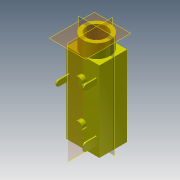
# Autodesk Inventor part: MJ-4535-3
Saved by Autodesk Inventor 2015 SP1 (Build 190203100, 203)
## iProperties
Created: 2015-04-15
Part Number: MJ-4535-3
Material: ABS プラスチック
Document SubType Name: Modeling
Designer: Yamaura
Density: 1.06 g/cm^3
Appearance: 滑らか - 黄
Author: Yamaura
Autodesk Inventor part; units mm, degrees
sketch "スケッチ1" plane through (0, 0, 0) normal (0, 0, 1) x (1, 0, 0)
  circle A0 centre (0, 0) radius 2.5
  circle A1 centre (0, 0) radius 1.8
  dimension "d0" = 5
  dimension "d1" = 3.6
  constraints: 2 centre point, 1 coincident
  measures "d0" diameter of A0
  measures "d1" diameter of A1
extrude "押し出し1" add sketch "スケッチ1" against normal blind 2.5
sketch "スケッチ2" plane through (0, 0, -2.5) normal (0, 0, -1) x (-1, 0, 0)
  line L0 (-3, 2.5) -> (3, 2.5)
  line L1 (3, 2.5) -> (3, -2.5)
  line L2 (3, -2.5) -> (-3, -2.5)
  line L3 (-3, -2.5) -> (-3, 2.5)
  point P0 (0, 0)
  dimension "d4" = 2.5
  dimension "d5" = 5
  dimension "d6" = 3
  dimension "d7" = 6
  constraints: 8 end point, 2 parallel, 1 horizontal, 1 perpendicular
  measures "d4" distance from line of L2 point (0, 0)
  measures "d5" distance of L2.end L0.start
  measures "d6" distance from line of L3 point (0, 0)
  measures "d7" distance of L0.start L0.end
extrude "押し出し2" add sketch "スケッチ2" along normal blind 14.5
sketch "スケッチ3" plane through (-3, -2.5, -2.5) normal (0, -1, 0) x (1, 0, 0)
  circle A0 centre (3, -3.6) radius 0.725
  line L0 (3, 0) -> (6, 0) projected
  circle A1 centre (3, -10.6) radius 0.725
  point P0 (3, 2.5)
  dimension "d10" = 1.45
  dimension "d11" = 3.6
  dimension "d12" = 1.45
  dimension "d13" = 7
  constraints: 2 centre point
  measures "d10" diameter of A0
  measures "d11" distance from line of L0 A0.centre
  measures "d12" diameter of A1
  measures "d13" distance of A1.centre A0.centre
extrude "押し出し3" add sketch "スケッチ3" along normal blind 0.8
sketch "スケッチ4" plane through (-3, -2.5, -2.5) normal (0, -1, 0) x (1, 0, 0)
  line L0 (5.35, -2.2) -> (5.55, -2.2)
  line L1 (5.55, -2.2) -> (5.55, -3.2)
  line L2 (5.55, -3.2) -> (5.35, -3.2)
  line L3 (5.35, -3.2) -> (5.35, -2.2)
  line L4 (0.65, -4) -> (0.45, -4)
  line L5 (0.45, -4) -> (0.45, -5)
  line L6 (0.45, -5) -> (0.65, -5)
  line L7 (0.65, -5) -> (0.65, -4)
  circle A0 centre (3, -3.6) radius 0.725 projected
  point P0 (3, 2.5)
  dimension "d16" = 0.2
  dimension "d17" = 0.2
  dimension "d18" = 2.55
  dimension "d19" = 2.55
  dimension "d20" = 1.4
  dimension "d21" = 1.4
  dimension "d22" = 1
  dimension "d23" = 1
  constraints: 16 end point, 4 parallel, 2 horizontal, 2 perpendicular
  measures "d16" distance of L0.start L0.end
  measures "d17" distance of L4.start L4.end
  measures "d18" distance from line of L1 A0.centre
  measures "d19" distance from line of L5 A0.centre
  measures "d20" distance from line of L0 A0.centre
  measures "d21" distance from line of L6 A0.centre
  measures "d22" distance of L0.end L1.end
  measures "d23" distance of L4.end L5.end
extrude "押し出し4" add sketch "スケッチ4" along normal blind 2.4 contours L0 L1 L2 L3 | L7 L6 L5 L4
sketch "スケッチ5" plane through (-3, -2.5, -2.5) normal (0, -1, 0) x (1, 0, 0)
  circle A0 centre (3, -10.6) radius 0.725 projected
  line L0 (5.55, -2.2) -> (5.55, -3.2) projected
  line L1 (5.55, -3.2) -> (5.35, -3.2) projected
  line L2 (5.35, -3.2) -> (5.35, -2.2) projected
  line L3 (5.35, -2.2) -> (5.55, -2.2) projected
  line L4 (0.65, -4) -> (0.65, -5) projected
  line L5 (0.65, -5) -> (0.45, -5) projected
  line L6 (0.45, -5) -> (0.45, -4) projected
  line L7 (0.45, -4) -> (0.65, -4) projected
  circle A1 centre (3, -3.6) radius 0.725 projected
  circle A2 centre (3, -10.6) radius 0.725 projected
  line L8 (0, 0) -> (3, 0) projected
  line L9 (0, 0) -> (0, -14.5) projected
  line L10 (6, -14.5) -> (0, -14.5) projected
  line L11 (6, 0) -> (6, -14.5) projected
  line L12 (3, 0) -> (6, 0) projected
  line L13 (5.35, -11.3) -> (5.55, -11.3)
  line L14 (5.55, -11.3) -> (5.55, -12.8)
  line L15 (5.55, -12.8) -> (5.35, -12.8)
  line L16 (5.35, -12.8) -> (5.35, -11.3)
  point P0 (3, 2.5)
  dimension "d26" = 0.2
  dimension "d27" = 1.5
  dimension "d28" = 2.2
  dimension "d29" = 2.55
  constraints: 8 end point, 2 parallel, 1 horizontal, 1 perpendicular
  measures "d26" distance of L14.end L15.end
  measures "d27" distance of L13.end L14.end
  measures "d28" distance from line of L15 A0.centre
  measures "d29" distance from line of L14 A0.centre
extrude "押し出し5" add sketch "スケッチ5" along normal blind 2.4 contours L13 L14 L15 L16
fillet "フィレット1" radius 0.5 6 edges at (2.45, -4.9, -5.7) (2.45, -4.9, -4.7) (-2.45, -4.9, -6.5) (-2.45, -4.9, -7.5) (2.45, -4.9, -13.8) (2.45, -4.9, -15.3)
